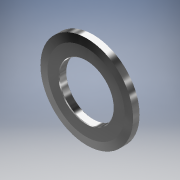
# Autodesk Inventor part: trim washer
Saved by Autodesk Inventor 2019 (Build 230136000, 136)
## iProperties
Shininess: 86.0
Length Units: 11272
Angle Units: 11279
Time Units: 11290
Mass Units: 11286
Length Display Precision: 3
Angle Display Precision: 2
Compacted: True
Created: 2001-07-10
Part Number: trim washer
Document SubType Name: Modeling
Designer: Autodesk, Inc.
Mass: 2.31528 g
Surface Area: 5.06704 cm^2
Volume: 0.286544 cm^3
Density: 8.08 g/cm^3
Material: Stainless Steel
Appearance: Chrome - Polished
Density: 0.0
Volumn: 0.0
Area: 0.0
PropertySet Name: Model Information
Control State: 0
Master: False
Checked Out: False
Author: Autodesk, Inc.
Autodesk Inventor part; units mm, degrees
ref_plane "YZ Plane" through (0, 0, 0) normal (1, 0, 0) x (0, 1, 0)
ref_plane "XZ Plane" through (0, 0, 0) normal (0, 1, 0) x (-1, 0, 0)
ref_plane "XY Plane" through (0, 0, 0) normal (0, 0, 1) x (1, 0, 0)
sketch "Sketch1" plane through (0, 0, 0) normal (0, 0, 1) x (1, 0, 0)
  circle A0 centre (0, 0) radius 5.5563
  circle A1 centre (0, 0) radius 9.525
  dimension "d0" = 11.1125
  constraints: 2 centre point, 1 coincident
  measures "d0" diameter of A0
extrude "Extrusion1" add sketch "Sketch1" along normal blind 1.5875
chamfer "Chamfer1" distance 0.127 distance2 1.5875 1 edges at (-9.525, 0, 1.5875) measured on face at (9.4941, -0.7664, 1.0583)
chamfer "Chamfer2" distance 1.5875 distance2 0.127 1 edges at (-9.525, 0, 0) measured on face at (8.1098, -0.7598, 0)
chamfer "Chamfer3" distance 0.127 angle 45 2 edges at (-5.5563, 0, 0) (-5.5563, 0, 1.5875)
body "Solid1"
